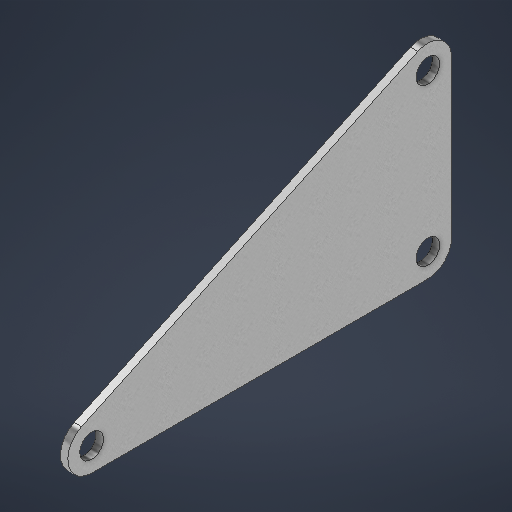
# Autodesk Inventor part: RockerFront
Saved by Autodesk Inventor 2026.2 (Build 302298010, 298A)
## iProperties
Created: 2026-08-01
Part Number: RockerFront
Material: Generic
Document SubType Name: Modeling
Designer: tasle
Density: 1 g/cm^3
Appearance: Default
Mass: 13.4289 g
Surface Area: 117.851 cm^2
Volume: 13.4289 cm^3
Author: tasle
Autodesk Inventor part; units mm, degrees
ref_plane "YZ Plane" through (0, 0, 0) normal (1, 0, 0) x (0, 1, 0)
ref_plane "XZ Plane" through (0, 0, 0) normal (0, 1, 0) x (-1, 0, 0)
ref_plane "XY Plane" through (0, 0, 0) normal (0, 0, 1) x (1, 0, 0)
sketch "Sketch1" plane through (0, 0, 0) normal (1, 0, 0) x (0, 1, 0)
  line L0 (0, 0) -> (52.8273, -113.2885)
  line L1 (0, 0) -> (0, -113.2885)
  circle A0 centre (52.8273, -113.2885) radius 4
  circle A1 centre (0, 0) radius 4
  circle A2 centre (52.8273, -113.2885) radius 8
  circle A3 centre (0, 0) radius 8
  line L2 (60.0777, -109.9075) -> (7.2505, 3.3809)
  circle A4 centre (0, -113.2885) radius 8
  line L3 (-8, 0) -> (-8, -113.2885)
  line L4 (0, -121.2885) -> (52.8273, -121.2885)
  circle A5 centre (0, -113.2885) radius 4
  dimension "d0" = 125
  dimension "d1" = 25
  dimension "d2" = 8
  dimension "d3" = 8
  dimension "d4" = 16
  dimension "d5" = 16
  dimension "d6" = 16
  dimension "d7" = 8
  constraints: 10 end point, 6 centre point, 6 coincident, 6 point on circle, 2 tangent, 1 horizontal, 1 horizontal alignment, 1 parallel, 1 vertical
  measures "d0" distance of L0.start L0.end
  measures "d1" angle of L1 L0
  measures "d2" diameter of A0
  measures "d3" diameter of A1
  measures "d4" diameter of A2
  measures "d5" diameter of A3
  measures "d6" diameter of A4
  measures "d7" diameter of A5
extrude "Extrusion1" add sketch "Sketch1" along normal blind 2.5 contours A1 L1 A3 L0 | L0 A3 L1 A1 | A3 L2 A2 L0 | L0 A2 L4 A4 L1 A3 | L1 A4 L3 A3 | A2 | A4
body "Solid1"
